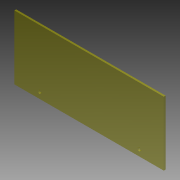
# Autodesk Inventor part: visor
Saved by Autodesk Inventor 2014 SP2 (Build 180246200, 246)
## iProperties
Created: 2016-05-05
Part Number: visor
Material: Generic
Document SubType Name: Modeling
Designer: cruiser
Density: 1 g/cm^3
Appearance: Clear - Yellow
Author: cruiser
Autodesk Inventor part; units mm, degrees
ref_plane "YZ Plane" through (0, 0, 0) normal (1, 0, 0) x (0, 1, 0)
ref_plane "XZ Plane" through (0, 0, 0) normal (0, 1, 0) x (-1, 0, 0)
ref_plane "XY Plane" through (0, 0, 0) normal (0, 0, 1) x (1, 0, 0)
sketch "Sketch1" plane through (0, 0, 0) normal (0, 1, 0) x (-1, 0, 0)
  line L0 (128.65, -55.1187) -> (-128.65, -55.1188)
  line L1 (-128.65, -55.1188) -> (-128.65, 55.1187)
  line L2 (-128.65, 55.1187) -> (128.65, 55.1188)
  line L3 (128.65, 55.1188) -> (128.65, -55.1187)
  line L4 (128.65, -55.1187) -> (-128.65, 55.1187) construction
  line L5 (-128.65, -55.1188) -> (128.65, 55.1188) construction
  point P0 (0, 0)
  dimension "d0" = 257.3
  dimension "d1" = 110.2375
  constraints: 12 end point, 2 midpoint, 2 parallel, 1 horizontal, 1 perpendicular
  measures "d0" distance of L1.end L2.end
  measures "d1" distance of L0.end L1.end
extrude "Extrusion1" add sketch "Sketch1" along normal blind 3.15
sketch "Sketch2" plane through (0, 3.15, 0) normal (0, 1, 0) x (1, 0, 0)
  line L0 (128.65, 55.1188) -> (-128.65, 55.1187) projected
  circle A0 centre (-85.7667, 45.1187) radius 2.5
  line L1 (0, 0) -> (0, 55.1188)
  circle A1 centre (85.7667, 45.1188) radius 2.5
  dimension "d4" = 5
  dimension "d5" = 10
  dimension "d6" = 85.7667
  constraints: 2 centre point, 2 end point, 1 midpoint, 1 symmetric about line, 1 other
  measures "d4" diameter of A0
  measures "d5" distance from line of L0 A0.centre
  measures "d6" distance from line of L1 A0.centre
extrude "Extrusion2" cut sketch "Sketch2" against normal blind 3.15
equation "\"d0\" = visor_x"
equation "\"d1\" = visor_y"
equation "\"d2\" = clear_acrylic"
equation "\"d4\" = m5_diameter"
equation "\"d5\" = 0.5 * visor_overlap"
equation "\"d6\" = 0.333333 * visor_x"
equation "\"d7\" = clear_acrylic"
equation "\"sm_thickness\" = 1.5875"
equation "\"very_thick_acrylic\" = 9.45"
equation "\"thick_acrylic\" = 5.88"
equation "\"thin_acrylic\" = 3.15"
equation "\"clear_acrylic\" = 3.15"
equation "\"wood_thickness\" = 6.72"
equation "\"m3_diameter\" = 3"
equation "\"m4_diameter\" = 4"
equation "\"m5_diameter\" = 5"
equation "\"brass_insert_drill\" = 4"
equation "\"m5_brass_insert_drill\" = 6.7"
equation "\"m3_main_length\" = 14"
equation "\"m3_main_nut_width\" = 5.7"
equation "\"m3_main_nut_thickness\" = 2.5"
equation "\"m3_main_extra\" = 1"
equation "\"stepper_screw_space\" = 35"
equation "\"stepper_shaft_diameter\" = 5"
equation "\"stepper_body_diameter\" = 28"
equation "\"laser_body_diameter\" = 12"
equation "\"t_carrier\" = 5.88"
equation "\"t_wall\" = 5.88"
equation "\"t_window\" = 3.15"
equation "\"carrier_y\" = 251"
equation "\"carrier_z\" = 12"
equation "\"carrier_z2\" = 328.24"
equation "\"protection_slot\" = 44.2"
equation "\"protection_slot_offset\" = 55.25"
equation "\"window_z\" = 334.9125"
equation "\"window_y\" = 92.0625"
equation "\"door_sensor\" = 35"
equation "\"reservoir_x\" = 201"
equation "\"reservoir_y\" = 201"
equation "\"linear_bearing_spacing\" = 271"
equation "\"motor_spacing\" = 337"
equation "\"t_tray\" = 3.15"
equation "\"tray_border\" = 25"
equation "\"tray_x\" = 251"
equation "\"tray_y\" = 251"
equation "\"bed_z\" = 25.4"
equation "\"bed_z2\" = 79.6"
equation "\"brass_keep_out\" = 8"
equation "\"tape_keep_out\" = 2"
equation "\"tape_thickness\" = 2"
equation "\"t_crane\" = 6.72"
equation "\"crane_z2\" = 12"
equation "\"end_stop_spacing\" = 19"
equation "\"thumb_nut_offset_y\" = 0"
equation "\"thumb_nut_diameter\" = 7"
equation "\"z_min_from_center\" = 115"
equation "\"t_frame\" = 6.72"
equation "\"frame_top_z\" = 386"
equation "\"frame_bottom_z\" = 275"
equation "\"frame_total_z\" = 661"
equation "\"frame_border\" = 46.35"
equation "\"frame_foot_z\" = 12"
equation "\"frame_tilt\" = 1deg"
equation "\"printer_z\" = 289"
equation "\"lcd_x\" = 72"
equation "\"lcd_y\" = 25"
equation "\"subframe_x\" = 195"
equation "\"subframe_y_offset\" = 27.5"
equation "\"laser_y_offset\" = 19.4"
equation "\"laser_diameter\" = 12"
equation "\"laser_z_offset\" = 55"
equation "\"laser_y\" = 35"
equation "\"laser_z\" = 18"
equation "\"laser_x\" = 24"
equation "\"t_galvo_frame\" = 6.72"
equation "\"galvo_frame_x\" = 66"
equation "\"galvo_frame_z\" = 65"
equation "\"galvo_frame_y_offset\" = 27.5"
equation "\"drawer_x\" = 257.3"
equation "\"drawer_y\" = 88.65"
equation "\"drawer_z\" = 278.175"
equation "\"drawer_z_from_bottom\" = 25"
equation "\"nema17_x\" = 43"
equation "\"visor_y\" = 110.2375"
equation "\"visor_x\" = 257.3"
equation "\"door_z\" = 334.9125"
equation "\"door_x\" = 251"
equation "\"window_overlap\" = 47.4675"
equation "\"door_overlap\" = 47.4675"
equation "\"acrylic_into_frame\" = 5"
equation "\"m3_press_nut_drill\" = 4.5"
equation "\"m3_head\" = 6"
equation "\"m5_press_nut_drill\" = 6.5"
equation "\"drawer_support_from_top\" = 47.4675"
equation "\"visor_overlap\" = 20"
body "Solid1"
